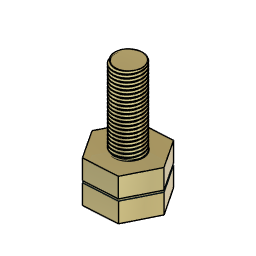
jaaaaaaaaaaaaduuuuuuuuuu (Autodesk Fusion 360 design; units mm, degrees)
Autodesk Fusion 360 part; units mm, degrees
sketch "Sketch1" plane through (0, 0, 0) normal (0, 0, 1) x (1, 0, 0)
  circle A0 centre (0, 0) radius 15
  line L0 (34.6371, 0.5196) -> (16.8686, 30.2564)
  line L1 (16.8686, 30.2564) -> (-17.7685, 29.7368)
  line L2 (-17.7685, 29.7368) -> (-34.6371, -0.5196)
  line L3 (-34.6371, -0.5196) -> (-16.8686, -30.2564)
  line L4 (-16.8686, -30.2564) -> (17.7685, -29.7368)
  line L5 (17.7685, -29.7368) -> (34.6371, 0.5196)
  dimension "d1" = 30
  dimension "d2" = 30
  constraint coincident A0.centre origin
  measures "d1" diameter of A0
  measures "d2" distance of A0.centre L5
extrude "Extrude1" add sketch "Sketch1" along normal blind 20 makes body 1
sketch "Sketch2" plane through (0, 0, 0) normal (0, 0, 1) x (1, 0, 0)
  line L0 (184.5696, 2.2237) -> (165.359, 31.05)
  line L1 (165.359, 31.05) -> (130.7895, 28.8263)
  line L2 (130.7895, 28.8263) -> (115.4304, -2.2237)
  line L3 (115.4304, -2.2237) -> (134.641, -31.05)
  line L4 (134.641, -31.05) -> (169.2105, -28.8263)
  line L5 (169.2105, -28.8263) -> (184.5696, 2.2237)
  point P0 (150, 0)
  dimension "d5" = 30
  measures "d5" distance of P0 L5
extrude "Extrude2" add sketch "Sketch2" along normal blind 20 separate body makes body 2
sketch "Sketch3" plane through (0, 0, 20) normal (0, 0, 1) x (-1, 0, 0)
  line L0 (-169.2105, 28.8263) -> (-184.5696, -2.2237)
  line L1 (-184.5696, -2.2237) -> (-165.359, -31.05)
  line L2 (-165.359, -31.05) -> (-130.7895, -28.8263)
  line L3 (-130.7895, -28.8263) -> (-115.4304, 2.2237)
  line L4 (-115.4304, 2.2237) -> (-134.641, 31.05)
  line L5 (-134.641, 31.05) -> (-169.2105, 28.8263)
sketch "Sketch4" plane through (0, 0, 20) normal (0, 0, 1) x (-1, 0, 0)
  circle A0 centre (-150, 0) radius 15
  dimension "d8" = 30
  measures "d8" diameter of A0
extrude "Extrude3" add sketch "Sketch4" along normal blind 100 bodies 2
thread "Thread1" "ISO Metric profile 30.0 M30x3.5 M30x3.5 6g" major diameter 29.7345 minor diameter 25.732 pitch 3.5 angle 60 modelled right hand crest width 0.4992 on face at (135.0745, 1.4935, 53.3333) crest through (135.1327, 0, 19.125) on bodies 2
thread "Thread2" "ISO Metric profile 30.0 M30x3.5 M30x3.5 6H" major diameter 30.3925 minor diameter 26.491 pitch 3.5 angle 60 modelled right hand crest width 0.9556 on face at (14.9814, -0.7477, 13.3333) crest through (13.2455, 0, 0.875) on bodies 1
copy_body "Body->Comp1" bodies 1 removing the originals makes body 3 in component "new model nut"
component "new model nut" placed x (-0.995307, 0.096763, 0) y (-0.096763, -0.995307, 0) z (0, 0, 1) at (150, 0, 25.0355)
named bodies: "new model nut", "new model bolt"
